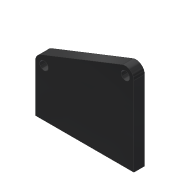
# Autodesk Inventor part: COXA_ROLL_COUPLER_BACK
Saved by Autodesk Inventor 2019.4 (Build 234330000, 330)
## iProperties
Created: 2019-10-21
Part Number: COXA_ROLL_COUPLER_BACK
Material: 一般
Document SubType Name: Modeling
Designer: y6tada
Density: 1 g/cm^3
Appearance: 濃い灰色
Author: y6tada
Autodesk Inventor part; units mm, degrees
ref_plane "YZ Plane" through (0, 0, 0) normal (1, 0, 0) x (0, 1, 0)
ref_plane "XZ Plane" through (0, 0, 0) normal (0, 1, 0) x (-1, 0, 0)
ref_plane "XY Plane" through (0, 0, 0) normal (0, 0, 1) x (1, 0, 0)
sketch "スケッチ1" plane through (0, 0, 0) normal (0, 0, 1) x (1, 0, 0)
  line L0 (0, 0) -> (38, 14.94) construction
  line L1 (36.5364, 18.6626) -> (-1.4636, 3.7226)
  line L2 (-4, 0) -> (-4, -22.2053)
  line L3 (-4, -22.2053) -> (42, -22.2053)
  line L4 (42, -22.2053) -> (42, 14.94)
  arc A0 (-1.4636, 3.7226) -> (-4, 0) centre (0, 0) ccw
  arc A1 (42, 14.94) -> (36.5364, 18.6626) centre (38, 14.94) ccw
  dimension "d0" = 38
  dimension "d1" = 14.94
  dimension "d2" = 4
  constraints: 10 end point, 4 coincident, 4 point on circle, 4 tangent, 2 centre point, 2 perpendicular, 1 equal radius, 1 horizontal
  measures "d0" horizontal distance of L0.end point (0, 0)
  measures "d1" vertical distance of point (0, 0) L0.end
  measures "d2" radius of A0
extrude "押し出し1" add sketch "スケッチ1" along normal blind 5
hole "穴1" at (0, 0, 0) at (38, 14.94, 0) direction (0, 0, 1) diameter 4 end through all
